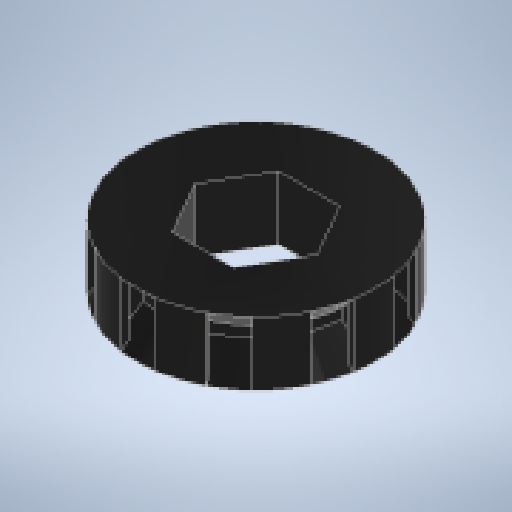
# Autodesk Inventor part: Tire Hub
Saved by Autodesk Inventor 2023.2 (Build 272271000, 271)
## iProperties
Created: 2023-02-06
Part Number: Tire Hub
Material: Nylon 6/6
Document SubType Name: Modeling
Designer: Nathan Cai
Density: 1.13 g/cm^3
Appearance: Smooth - Black
Mass: 3.14977 g
Surface Area: 28.8521 cm^2
Volume: 2.7874 cm^3
Wheel_OD: 1.250 in
Author: Nathan Cai
Autodesk Inventor part; units mm, degrees
ref_plane "YZ Plane" through (0, 0, 0) normal (1, 0, 0) x (0, 1, 0)
ref_plane "XZ Plane" through (0, 0, 0) normal (0, 1, 0) x (-1, 0, 0)
sketch "Sketch10" plane through (0, 0, 0) normal (0, 1, 0) x (-1, 0, 0)
  circle A0 centre (0, 0) radius 15.875 construction
  line L0 (0, 0) -> (15.875, 0) construction
  line L1 (7.3323, 0) -> (3.6662, -6.35)
  line L2 (3.6662, -6.35) -> (-3.6662, -6.35)
  line L3 (-3.6662, -6.35) -> (-7.3323, 0)
  line L4 (-7.3323, 0) -> (-3.6662, 6.35)
  line L5 (-3.6662, 6.35) -> (3.6662, 6.35)
  line L6 (3.6662, 6.35) -> (7.3323, 0)
  circle A1 centre (0, 0) radius 11.1125
  arc A2 (14.0704, -2.481) -> (14.0704, 2.481) centre (0, 0) ccw
  arc A3 (13.2887, -2.3432) -> (13.2887, 2.3432) centre (0, 0) ccw
  line L7 (11.0841, 0.7937) -> (13.4704, 0.7937)
  line L8 (14.251, 9.5243) -> (14.251, -1.0205) construction
  line L9 (13.4704, -0.7937) -> (11.0841, -0.7937)
  line L10 (13.2887, 2.3432) -> (14.0704, 2.481)
  line L11 (13.2887, -2.3432) -> (14.0704, -2.481)
  line L12 (8.5007, 7.1572) -> (10.4312, 8.5599)
  line L13 (11.3643, 7.2755) -> (9.4338, 5.8729)
  line L14 (9.3735, 9.7066) -> (9.9249, 10.2776)
  arc A4 (12.1281, 5.9153) -> (9.3735, 9.7066) centre (0, 0) ccw
  line L15 (5.9311, 16.0818) -> (12.1292, 7.5509) construction
  line L16 (12.1281, 5.9153) -> (12.8415, 6.2632)
  arc A5 (12.8415, 6.2632) -> (9.9249, 10.2776) centre (0, 0) ccw
  line L17 (2.6703, 10.7869) -> (3.4077, 13.0564)
  line L18 (4.9175, 12.5658) -> (4.1801, 10.2963)
  line L19 (1.878, 13.3624) -> (1.9884, 14.1485)
  arc A6 (6.3349, 11.9143) -> (1.878, 13.3624) centre (0, 0) ccw
  line L20 (-4.6543, 16.4967) -> (5.3744, 13.2381) construction
  line L21 (6.3349, 11.9143) -> (6.7076, 12.6151)
  arc A7 (6.7076, 12.6151) -> (1.9884, 14.1485) centre (0, 0) ccw
  line L22 (-4.1801, 10.2963) -> (-4.9175, 12.5658)
  line L23 (-3.4077, 13.0564) -> (-2.6703, 10.7869)
  line L24 (-6.3349, 11.9143) -> (-6.7076, 12.6151)
  arc A8 (-1.878, 13.3624) -> (-6.3349, 11.9143) centre (0, 0) ccw
  line L25 (-13.4619, 10.6103) -> (-3.4332, 13.8689) construction
  line L26 (-1.878, 13.3624) -> (-1.9884, 14.1485)
  arc A9 (-1.9884, 14.1485) -> (-6.7076, 12.6151) centre (0, 0) ccw
  line L27 (-9.4338, 5.8729) -> (-11.3643, 7.2755)
  line L28 (-10.4312, 8.5599) -> (-8.5007, 7.1572)
  line L29 (-12.1281, 5.9153) -> (-12.8415, 6.2632)
  arc A10 (-9.3735, 9.7066) -> (-12.1281, 5.9153) centre (0, 0) ccw
  line L30 (-17.1275, 0.6712) -> (-10.9294, 9.2022) construction
  line L31 (-9.3735, 9.7066) -> (-9.9249, 10.2776)
  arc A11 (-9.9249, 10.2776) -> (-12.8415, 6.2632) centre (0, 0) ccw
  line L32 (-11.0841, -0.7938) -> (-13.4704, -0.7937)
  line L33 (-13.4704, 0.7937) -> (-11.0841, 0.7937)
  line L34 (-13.2887, -2.3432) -> (-14.0704, -2.481)
  arc A12 (-13.2887, 2.3432) -> (-13.2887, -2.3432) centre (0, 0) ccw
  line L35 (-14.251, -9.5243) -> (-14.251, 1.0205) construction
  line L36 (-13.2887, 2.3432) -> (-14.0704, 2.481)
  arc A13 (-14.0704, 2.481) -> (-14.0704, -2.481) centre (0, 0) ccw
  line L37 (-8.5007, -7.1572) -> (-10.4312, -8.5599)
  line L38 (-11.3643, -7.2755) -> (-9.4338, -5.8729)
  line L39 (-9.3735, -9.7066) -> (-9.9249, -10.2776)
  arc A14 (-12.1281, -5.9153) -> (-9.3735, -9.7066) centre (0, 0) ccw
  line L40 (-5.9311, -16.0818) -> (-12.1292, -7.5509) construction
  line L41 (-12.1281, -5.9153) -> (-12.8415, -6.2632)
  arc A15 (-12.8415, -6.2632) -> (-9.9249, -10.2776) centre (0, 0) ccw
  line L42 (-2.6703, -10.7869) -> (-3.4077, -13.0564)
  line L43 (-4.9175, -12.5658) -> (-4.1801, -10.2963)
  line L44 (-1.878, -13.3624) -> (-1.9884, -14.1485)
  arc A16 (-6.3349, -11.9143) -> (-1.878, -13.3624) centre (0, 0) ccw
  line L45 (4.6543, -16.4967) -> (-5.3744, -13.2381) construction
  line L46 (-6.3349, -11.9143) -> (-6.7076, -12.6151)
  arc A17 (-6.7076, -12.6151) -> (-1.9884, -14.1485) centre (0, 0) ccw
  line L47 (4.1801, -10.2963) -> (4.9175, -12.5658)
  line L48 (3.4077, -13.0564) -> (2.6703, -10.7869)
  line L49 (6.3349, -11.9143) -> (6.7076, -12.6151)
  arc A18 (1.878, -13.3624) -> (6.3349, -11.9143) centre (0, 0) ccw
  line L50 (13.4619, -10.6103) -> (3.4332, -13.8689) construction
  line L51 (1.878, -13.3624) -> (1.9884, -14.1485)
  arc A19 (1.9884, -14.1485) -> (6.7076, -12.6151) centre (0, 0) ccw
  line L52 (9.4338, -5.8729) -> (11.3643, -7.2755)
  line L53 (10.4312, -8.5599) -> (8.5007, -7.1572)
  line L54 (12.1281, -5.9153) -> (12.8415, -6.2632)
  arc A20 (9.3735, -9.7066) -> (12.1281, -5.9153) centre (0, 0) ccw
  line L55 (17.1275, -0.6712) -> (10.9294, -9.2022) construction
  line L56 (9.3735, -9.7066) -> (9.9249, -10.2776)
  arc A21 (9.9249, -10.2776) -> (12.8415, -6.2632) centre (0, 0) ccw
  point P0 (9.4338, 5.8729)
  point P1 (8.5007, 7.1572)
  point P2 (4.1801, 10.2963)
  point P3 (2.6703, 10.7869)
  point P4 (-2.6703, 10.7869)
  point P5 (-4.1801, 10.2963)
  point P6 (-8.5007, 7.1572)
  point P7 (-9.4338, 5.8729)
  point P8 (-11.0841, 0.7937)
  point P9 (-9.4338, -5.8729)
  point P10 (-8.5007, -7.1572)
  point P11 (-4.1801, -10.2963)
  point P12 (-2.6703, -10.7869)
  point P13 (2.6703, -10.7869)
  point P14 (4.1801, -10.2963)
  point P15 (8.5007, -7.1572)
  dimension "Wheel_OD" = 31.75
  dimension "d65" = 12.7
  dimension "d66" = 22.225
  dimension "d67" = 28.575
  dimension "d68" = 0.7937
  dimension "d69" = 1.5875
  dimension "d71" = 10
  dimension "d74" = 360
  constraints: 114 end point, 72 point on circle, 21 centre point, 21 point on line, 15 coincident, 2 horizontal, 1 horizontal alignment, 1 parallel, 1 perpendicular, 216 other
  measures "d65" distance between parallel lines of L5 L2
  measures "d66" diameter of A1
  measures "d67" diameter of A2
  measures "d68" radial gap between concentric circles of A2 A3
  measures "d69" distance between parallel lines of L7 L9
  measures "d71" angle of L9 L11
extrude "Extrusion7" add sketch "Sketch10" along normal blind 7.62 contours A1
sketch "Sketch11" plane through (0, 7.62, 0) normal (0, 1, 0) x (1, 0, 0)
  circle A0 centre (0, 0) radius 14.2875
  circle A1 centre (0, 0) radius 11.1125
  dimension "d78" = 28.575
  dimension "d79" = 22.225
  constraints: 2 centre point, 2 coincident
  measures "d78" diameter of A0
  measures "d79" diameter of A1
extrude "Extrusion8" add sketch "Sketch11" against normal blind 3.175
chamfer "Chamfer5" distance 3.175 angle 45 1 edges at (-14.2875, 4.445, 0)
ref_plane "Work Plane4" through (0, 3.81, 0) normal (0, -1, 0) x (1, 0, 0)
mirror "Mirror2" about plane through (0, 3.81, 0) normal (0, -1, 0) of "Extrusion8", "Chamfer5"
extrude "Extrusion9" add sketch "Sketch10" along normal up to surface (7.62 mm away) contours A1 L7 A3 L9 | A1 L12 A4 L13 | A3 L10 A2 L11 | L52 A20 L53 A1 | A4 L14 A5 L16 | A20 L54 A21 L56 | A1 L17 A6 L18 | L47 A18 L48 A1 | A6 L19 A7 L21 | A18 L49 A19 L51 | A1 L22 A8 L23 | L42 A16 L43 A1 | A8 L24 A9 L26 | A16 L44 A17 L46 | A1 L27 A10 L28 | L37 A14 L38 A1 | A10 L29 A11 L31 | A14 L39 A15 L41 | A1 L32 A12 L33 | A12 L34 A13 L36
sketch "Sketch13" plane through (0, 0, 0) normal (1, 0, 0) x (0, 1, 0)
  line L0 (0, 0) -> (0, 6.35) projected
  line L1 (0, -14.1485) -> (0, -12.6151) projected
  line L2 (0, 0) -> (0, -14.1485)
  line L3 (0, -6.35) -> (0, 0) projected
  circle A0 centre (0, -11.1125) radius 1.5875
  line L4 (0, -2.481) -> (0, 2.481) projected
  line L5 (0, 0) -> (-10.6988, 0) construction
  dimension "d91" = 3.175
  dimension "d92" = 11.1125
  constraints: 4 end point, 1 centre point, 1 horizontal, 1 midpoint, 1 point on line, 1 vertical
  measures "d91" diameter of A0
  measures "d92" distance of L5.start A0.centre
revolve "Revolution2" cut sketch "Sketch13" angle 360 about axis through (0, 0, 0) along (0, -1, 0)
body "Solid2"
